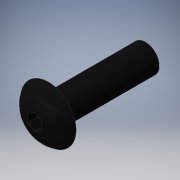
# Autodesk Inventor part: 14-20Bolt
Saved by Autodesk Inventor 2016 (Build 200138000, 138)
## iProperties
Created: 2017-01-15
Part Number: 14-20Bolt
Material: Steel, Galvanized
Document SubType Name: Modeling
Designer: Kyle
Density: 7.85 g/cm^3
Appearance: Glossy - Black
Mass: 7.22707 g
Surface Area: 7.70392 cm^2
Volume: 0.920646 cm^3
Author: Kyle
Autodesk Inventor part; units mm, degrees
ref_plane "YZ Plane" through (0, 0, 0) normal (1, 0, 0) x (0, 1, 0)
ref_plane "XZ Plane" through (0, 0, 0) normal (0, 1, 0) x (-1, 0, 0)
ref_plane "XY Plane" through (0, 0, 0) normal (0, 0, 1) x (1, 0, 0)
sketch "Sketch1" plane through (0, 0, 0) normal (0, 1, 0) x (-1, 0, 0)
  line L0 (0, 0) -> (0, -25.4)
  line L1 (0, -25.4) -> (3.175, -25.4)
  line L2 (3.175, -25.4) -> (3.175, -3.175)
  line L3 (3.175, -3.175) -> (6.35, -3.175)
  arc A0 (6.35, -3.175) -> (0, 0) centre (0.8204, -6.2968) ccw
  dimension "d0" = 25.4
  dimension "d1" = 3.175
  dimension "d2" = 22.225
  dimension "d3" = 3.175
  dimension "d4" = 6.35
  constraints: 8 end point, 3 perpendicular, 2 point on circle, 1 centre point, 1 vertical
  measures "d0" distance of L0.start L0.end
  measures "d1" distance of L0.end L1.end
  measures "d2" distance of L1.end L2.end
  measures "d3" distance of L2.end L3.end
  measures "d4" radius of A0
revolve "Revolution1" add sketch "Sketch1" angle 360 about axis through (0, 0, 0) along (0, 0, -1)
sketch "Sketch2" plane through (0, 0, -25.4) normal (0, 0, -1) x (-1, 0, 0)
  line L0 (-1.5875, 0.9165) -> (0, 1.8331)
  line L1 (0, 1.8331) -> (1.5875, 0.9165)
  line L2 (1.5875, 0.9165) -> (1.5875, -0.9165)
  line L3 (1.5875, -0.9165) -> (0, -1.8331)
  line L4 (0, -1.8331) -> (-1.5875, -0.9165)
  line L5 (-1.5875, -0.9165) -> (-1.5875, 0.9165)
  point P0 (0, 0)
  point P1 (0, 0)
  dimension "d7" = 3.175
  constraints: 12 end point, 1 coincident, 13 other
  measures "d7" distance between parallel lines of L5 L2
extrude "Extrusion1" cut sketch "Sketch2" against normal blind 31.75
sketch "Sketch3" plane through (0, 0, -25.4) normal (0, 0, -1) x (-1, 0, 0)
  line L0 (-1.5875, 0.9165) -> (0, 1.8331) projected
  line L1 (0, 1.8331) -> (1.5875, 0.9165) projected
  line L2 (1.5875, 0.9165) -> (1.5875, -0.9165) projected
  line L3 (1.5875, -0.9165) -> (0, -1.8331) projected
  line L4 (0, -1.8331) -> (-1.5875, -0.9165) projected
  line L5 (-1.5875, -0.9165) -> (-1.5875, 0.9165) projected
  point P0 (0, 0)
extrude "Extrusion2" add sketch "Sketch3" against normal blind 22.225
body "Solid1"
